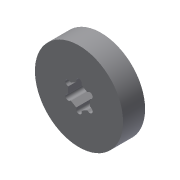
# Autodesk Inventor part: augmented gear
Saved by Autodesk Inventor 2014 (Build 180170000, 170)
## iProperties
Created: 2014-02-23
Part Number: augmented gear
Material: Generic
Document SubType Name: Modeling
Designer: Owner
Density: 1 g/cm^3
Appearance: Default
Author: Owner
Autodesk Inventor part; units mm, degrees
ref_plane "YZ Plane" through (0, 0, 0) normal (1, 0, 0) x (0, 1, 0)
ref_plane "XZ Plane" through (0, 0, 0) normal (0, 1, 0) x (-1, 0, 0)
ref_plane "XY Plane" through (0, 0, 0) normal (0, 0, 1) x (1, 0, 0)
sketch "Sketch1" plane through (0, 0, 0) normal (0, 0, 1) x (1, 0, 0)
  line L0 (7.9214, 13.0109) -> (7.9214, 20.2626) construction
  line L1 (7.9214, 13.0109) -> (14.2016, 16.6367) construction
  circle A0 centre (7.9214, 13.0109) radius 6.35 construction
  line L2 (7.9214, 13.0109) -> (14.2016, 9.385) construction
  line L3 (7.9214, 13.0109) -> (7.9214, 5.7592) construction
  line L4 (7.9214, 13.0109) -> (1.6413, 9.385) construction
  line L5 (7.9214, 13.0109) -> (1.6413, 16.6367) construction
  line L6 (7.9214, 20.2626) -> (14.2016, 16.6367)
  line L7 (14.2016, 16.6367) -> (14.2016, 9.385)
  line L8 (7.9214, 5.7592) -> (14.2016, 9.385)
  line L9 (7.9214, 5.7592) -> (1.6413, 9.385)
  line L10 (1.6413, 9.385) -> (1.6413, 16.6367)
  line L11 (1.6413, 16.6367) -> (7.9214, 20.2626)
  circle A1 centre (7.9214, 13.0109) radius 25.4
  circle A2 centre (7.9214, 20.2626) radius 1.5875
  circle A3 centre (14.2016, 16.6367) radius 1.5875
  circle A4 centre (14.2016, 9.385) radius 1.5875
  circle A5 centre (7.9214, 5.7592) radius 1.5875
  circle A6 centre (1.6413, 9.385) radius 1.5875
  circle A7 centre (1.6413, 16.6367) radius 1.5875
  line L12 (6.3339, 20.2626) -> (9.5089, 20.2626)
  line L13 (9.5089, 20.2626) -> (9.5089, 19.346)
  line L14 (9.5089, 19.346) -> (6.3339, 19.346)
  line L15 (6.3339, 19.346) -> (6.3339, 20.2626)
  line L16 (12.6141, 8.4685) -> (13.4078, 8.0102)
  line L17 (13.4078, 8.0102) -> (14.9953, 10.7598)
  line L18 (14.9953, 10.7598) -> (14.2016, 11.2181)
  line L19 (14.2016, 11.2181) -> (12.6141, 8.4685)
  line L20 (6.3339, 6.6757) -> (6.3339, 5.7592)
  line L21 (6.3339, 5.7592) -> (9.5089, 5.7592)
  line L22 (9.5089, 5.7592) -> (9.5089, 6.6757)
  line L23 (9.5089, 6.6757) -> (6.3339, 6.6757)
  line L24 (1.6413, 11.2181) -> (0.8475, 10.7598)
  line L25 (0.8475, 10.7598) -> (2.435, 8.0102)
  line L26 (2.435, 8.0102) -> (3.2288, 8.4685)
  line L27 (3.2288, 8.4685) -> (1.6413, 11.2181)
  line L28 (3.2288, 17.5532) -> (2.435, 18.0115)
  line L29 (2.435, 18.0115) -> (0.8475, 15.2619)
  line L30 (0.8475, 15.2619) -> (1.6413, 14.8036)
  line L31 (1.6413, 14.8036) -> (3.2288, 17.5532)
  line L32 (14.2016, 14.8036) -> (14.9953, 15.2619)
  line L33 (14.9953, 15.2619) -> (13.4078, 18.0115)
  line L34 (13.4078, 18.0115) -> (12.6141, 17.5532)
  line L35 (12.6141, 17.5532) -> (14.2016, 14.8036)
  dimension "d9" = 3.175
  dimension "d11" = 3.175
  dimension "d0" = 7.2517
  dimension "d1" = 12.7
  dimension "d2" = 60
  dimension "d3" = 60
  dimension "d4" = 60
  dimension "d5" = 60
  dimension "d6" = 60
  dimension "d7" = 3.175
  dimension "d8" = 3.175
  dimension "d10" = 3.175
  dimension "d12" = 3.175
  dimension "d13" = 50.8
  dimension "d14" = 0.9165
  dimension "d16" = 0.9165
  dimension "d17" = 0.9165
  dimension "d18" = 0.9165
  dimension "d19" = 0.9165
  dimension "d20" = 0.9165
  constraints: 72 end point, 14 parallel, 8 coincident, 8 tangent, 7 point on line, 6 centre point, 6 perpendicular, 5 equal length, 2 horizontal, 1 vertical, 10 other
  measures "d0" distance of L0.start L0.end
  measures "d1" diameter of A0
  measures "d2" angle of L1 L0
  measures "d3" angle of L2 L1
  measures "d4" angle of L3 L2
  measures "d5" angle of L4 L3
  measures "d6" angle of L5 L4
  measures "d7" diameter of A2
  measures "d8" diameter of A3
  measures "d10" diameter of A5
  measures "d12" diameter of A7
  measures "d13" diameter of A1
  measures "d14" distance of L12.end L13.end
  measures "d16" distance of L16.start L16.end
  measures "d17" distance of L20.start L20.end
  measures "d18" distance of L25.end L26.end
  measures "d19" distance of L28.start L28.end
  measures "d20" distance of L32.start L32.end
extrude "Extrusion1" add sketch "Sketch1" against normal blind 12.7
equation "\"d9\" = d7"
equation "\"d11\" = d7"
equation "\"d8\" = d7"
equation "\"d10\" = d7"
equation "\"d12\" = d7"
body "Solid1"
